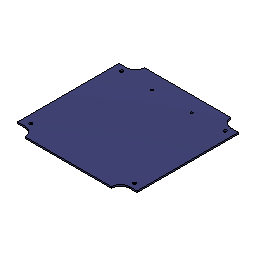
Electronics box v29_full (Autodesk Fusion 360 archive; units mm, degrees)
design "Node PCB DW"
Autodesk Fusion 360 part; units mm, degrees
sketch "Sketch1" plane through (0, 0, 0) normal (0, 1, 0) x (1, 0, 0)
  line L0 (50.25, 69.5) -> (-50.25, 69.5)
  line L1 (-69.5, 59) -> (-69.5, -59)
  line L2 (-50.25, -69.5) -> (50.25, -69.5)
  line L3 (69.5, -59) -> (69.5, 59)
  line L4 (-69.5, -59) -> (-60.75, -59)
  arc A0 (-50.25, -69.5) -> (-60.75, -59) centre (-60.75, -69.5) ccw
  circle A1 centre (-60.25, -52.75) radius 1.75
  line L5 (0, 69.5) -> (0, -69.5)
  line L6 (-69.5, 0) -> (69.5, 0)
  line L7 (69.5, -59) -> (60.75, -59)
  arc A2 (60.75, -59) -> (50.25, -69.5) centre (60.75, -69.5) ccw
  circle A3 centre (60.25, -52.75) radius 1.75
  arc A4 (50.25, 69.5) -> (60.75, 59) centre (60.75, 69.5) ccw
  line L8 (69.5, 59) -> (60.75, 59)
  circle A5 centre (60.25, 52.75) radius 1.75
  arc A6 (-60.75, 59) -> (-50.25, 69.5) centre (-60.75, 69.5) ccw
  line L9 (-69.5, 59) -> (-60.75, 59)
  circle A7 centre (-60.25, 52.75) radius 1.75
  circle A8 centre (-23.5, 51.5) radius 1.25
  circle A9 centre (22.5, 51.5) radius 1.25
  dimension "d5" = 10.5
  dimension "d7" = 50.25
  dimension "d8" = 59
  dimension "d9" = 69.5
  dimension "d10" = 69.5
  dimension "d11" = 3.5
  dimension "d12" = 52.75
  dimension "d13" = 60.25
  dimension "d14" = 69.5
  dimension "d15" = 139
  dimension "d16" = 2.5
  dimension "d19" = 18
  dimension "d22" = 46
  dimension "d23" = 2.5
  dimension "d24" = 46
  dimension "d25" = 47
  constraint horizontal L0
  constraint perpendicular L0 L1
  constraint parallel L0 L2
  constraint parallel L1 L3
  constraint perpendicular L3 L4
  constraint tangent L4 A0
  constraint coincident L2 L5.end
  constraint perpendicular L2 L5
  constraint coincident L1 L6.start
  constraint perpendicular L3 L6
  constraint symmetric L1.end L5 L3.start
  constraint symmetric L2.start L5 L2.end
  constraint symmetric L4.end L5 L7.end
  constraint symmetric A0 L5 A2
  constraint symmetric A1 L5 A3
  constraint symmetric L1.end L6 L1.start
  constraint symmetric L2.start L6 L0.end
  constraint symmetric L4.end L6 A6.start
  constraint symmetric A0 L6 A6
  constraint symmetric A1 L6 A7
  constraint symmetric L6 L3.start L3.end
  constraint symmetric L6 L7.end A4.end
  constraint symmetric L6 L2.end L0.start
  constraint symmetric L6 A2 A4
  constraint symmetric L6 A3 A5
  constraint coincident L0 L5.start
  constraint coincident L3 L6.end
  constraint horizontal A8.centre A9.centre
  measures "d5" radius of A0
  measures "d7" horizontal distance of origin L2.start
  measures "d8" vertical distance of origin L1.end
  measures "d9" distance of L2 origin
  measures "d10" distance of L1 origin
  measures "d11" diameter of A1
  measures "d12" vertical distance of origin A1.centre
  measures "d13" horizontal distance of origin A1.centre
  measures "d14" distance of L0 origin
  measures "d15" distance of L1 L3
  measures "d16" diameter of A8
  measures "d19" distance of L0 A8.centre
  measures "d22" distance of L1 A8.centre
  measures "d23" diameter of A9
  measures "d24" distance of A8.centre A9.centre
  measures "d25" distance of L3 A9.centre
extrude "Extrude1" add sketch "Sketch1" along normal blind 1.7
equation "d3 = 10.5 mm"
equation "d5 = d3"
equation "d12 = ( 105.5 / 2 ) * 1 mm"
equation "d13 = ( 120.5 / 2 ) * 1 mm"
equation "d22 = 44.75 mm + d16 / 2"
equation "d23 = d16"
